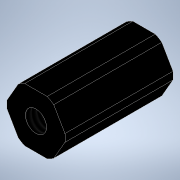
# Autodesk Inventor part: ThunderHex Shaft Creator
Saved by Autodesk Inventor 2022.3 (Build 263350000, 350)
## iProperties
Created: 2023-01-23
Part Number: ThunderHex Shaft Creator
Material: Aluminum 6061
Document SubType Name: Modeling
Designer: 23kaltomare
Density: 2.7 g/cm^3
Appearance: Anodized - Black
RuleStatus: InUse
AfterDocNew0: Rule0
Author: 23kaltomare
Autodesk Inventor part; units mm, degrees
ref_plane "YZ Plane" through (0, 0, 0) normal (1, 0, 0) x (0, 1, 0)
ref_plane "XZ Plane" through (0, 0, 0) normal (0, 1, 0) x (-1, 0, 0)
ref_plane "XY Plane" through (0, 0, 0) normal (0, 0, 1) x (1, 0, 0)
sketch "Sketch1" plane through (0, 0, 0) normal (0, 0, 1) x (1, 0, 0)
  line L0 (3.6662, -6.35) -> (-3.6662, -6.35)
  line L1 (-3.6662, -6.35) -> (-7.3323, 0)
  line L2 (-7.3323, 0) -> (-3.6662, 6.35)
  line L3 (-3.6662, 6.35) -> (3.6662, 6.35)
  line L4 (3.6662, 6.35) -> (7.3323, 0)
  line L5 (7.3323, 0) -> (3.6662, -6.35)
  circle A0 centre (0, 0) radius 6.875
  point P0 (2.635, -6.35)
  point P1 (4.1818, -5.457)
  point P2 (6.8168, -0.893)
  point P3 (6.8168, 0.893)
  point P4 (4.1818, 5.457)
  point P5 (2.635, 6.35)
  point P6 (-2.635, 6.35)
  point P7 (-4.1818, 5.457)
  point P8 (-6.8168, 0.893)
  point P9 (-6.8168, -0.893)
  point P10 (-4.1818, -5.457)
  point P11 (-2.635, -6.35)
  dimension "d0" = 12.7
  dimension "d1" = 13.75
  constraints: 12 end point, 2 coincident, 1 centre point, 1 horizontal, 13 other
  measures "d0" distance between parallel lines of L0 L3
  measures "d1" diameter of A0
extrude "Extrusion1" add sketch "Sketch1" along normal mid plane 25.4 contours L0 A0 L1 L2 L3 L4 L5
sketch "Sketch2" plane through (0, 0, 12.7) normal (0, 0, 1) x (1, 0, 0)
  point P0 (0, 0)
  point P1 (0, 0)
  constraints: 1 coincident
hole "Hole1" at (0, 0, 12.7) direction (0, 0, -1) diameter 4.9784 end through all thread size "1/4-20 UNC" class "2B" standard "ANSI Unified Screw Threads"
equation "\"d2\" = ShaftLength"
equation "\"ShaftLength\" = 25.4"
body "Solid1"
